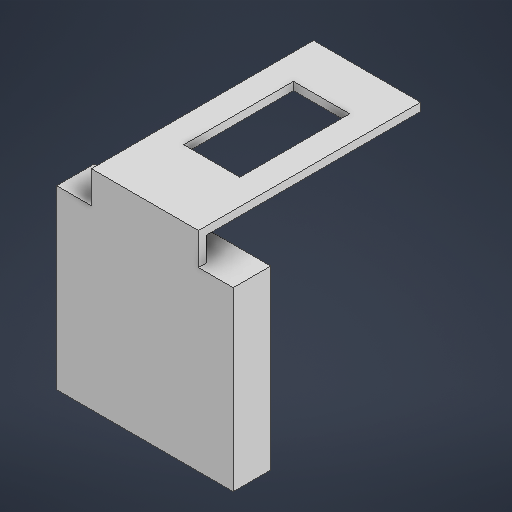
# Autodesk Inventor part: pan_base_holder
Saved by Autodesk Inventor 2026 (Build 300175000, 175)
## iProperties
Created: 2025-06-27
Part Number: pan_base_holder
Material: Generic
Document SubType Name: Modeling
Designer: user
Density: 1 g/cm^3
Appearance: Default
Author: user
Autodesk Inventor part; units mm, degrees
ref_plane "YZ Plane" through (0, 0, 0) normal (1, 0, 0) x (0, 1, 0)
ref_plane "XZ Plane" through (0, 0, 0) normal (0, 1, 0) x (-1, 0, 0)
ref_plane "XY Plane" through (0, 0, 0) normal (0, 0, 1) x (1, 0, 0)
sketch "Sketch1" plane through (0, 0, 0) normal (0, 0, 1) x (1, 0, 0)
  line L0 (-31, -31) -> (31, -31)
  line L1 (31, -31) -> (31, 31)
  line L2 (31, 31) -> (-31, 31)
  line L3 (-31, 31) -> (-31, -31)
  line L4 (-31, -31) -> (31, 31) construction
  line L5 (31, -31) -> (-31, 31) construction
  line L6 (-33, 33) -> (33, 33)
  line L7 (33, 33) -> (33, -33)
  line L8 (33, -33) -> (-33, -33)
  line L9 (-33, -33) -> (-33, 33)
  point P0 (0, 0)
  dimension "d0" = 62
  dimension "d1" = 62
  dimension "d2" = 2
  constraints: 20 end point, 4 parallel, 2 midpoint, 2 perpendicular, 1 horizontal, 3 other
  measures "d0" distance of L1.end L2.end
  measures "d1" distance of L0.end L1.end
  measures "d2" distance between parallel lines of L2 L6
extrude "Extrusion1" add sketch "Sketch1" along normal blind 2 contours L3 L2 L1 L0 | L6 L7 L8 L9
extrude "Extrusion2" add sketch "Sketch1" against normal blind 12
sketch "Sketch2" plane through (-33, 33, 2) normal (0, 1, 0) x (1, 0, 0)
  line L0 (13, 3) -> (53, 3)
  line L1 (53, 3) -> (53, 0)
  line L2 (53, 0) -> (13, 0)
  line L3 (13, 0) -> (13, 3)
  line L4 (0, 14) -> (0, 0) projected
  line L5 (0, 14) -> (66, 14) projected
  point P0 (33, 2)
  dimension "d7" = 40
  dimension "d8" = 3
  dimension "d9" = 13
  dimension "d10" = 11
  constraints: 8 end point, 2 parallel, 1 horizontal, 1 perpendicular
  measures "d7" distance of L1.end L2.end
  measures "d8" distance of L0.end L1.end
  measures "d9" distance between parallel lines of L4 L3
  measures "d10" distance between parallel lines of L5 L0
extrude "Extrusion3" add sketch "Sketch2" along normal blind 12
sketch "Sketch3" plane through (20, 33, -1) normal (0, 0, -1) x (-1, 0, 0)
  line L0 (40, 12) -> (0, 12) projected
  line L1 (40, 0) -> (40, 12) projected
  line L2 (0, 12) -> (40, 12)
  line L3 (40, 12) -> (40, 9)
  line L4 (40, 9) -> (0, 9)
  line L5 (0, 9) -> (0, 12)
  point P0 (20, -33)
  dimension "d13" = 3
  constraints: 8 end point, 2 parallel, 1 horizontal, 1 perpendicular, 1 point on line
  measures "d13" distance of L2.end L3.end
extrude "Extrusion4" add sketch "Sketch3" along normal blind 80
sketch "Sketch4" plane through (-20, 42, -1) normal (0, -1, 0) x (1, 0, 0)
  line L0 (30.5, -63) -> (9.5, -63)
  line L1 (9.5, -63) -> (9.5, -22)
  line L2 (9.5, -22) -> (30.5, -22)
  line L3 (30.5, -22) -> (30.5, -63)
  line L4 (40, 3) -> (40, -80) projected
  line L5 (0, 3) -> (40, 3) projected
  point P0 (20, 1)
  dimension "d16" = 21
  dimension "d17" = 41
  dimension "d18" = 9.5
  dimension "d19" = 25
  constraints: 8 end point, 2 parallel, 1 horizontal, 1 perpendicular
  measures "d16" distance of L0.start L0.end
  measures "d17" distance of L0.end L1.end
  measures "d18" distance between parallel lines of L4 L3
  measures "d19" distance between parallel lines of L2 L5
extrude "Extrusion5" cut sketch "Sketch4" against normal blind 80
body "Solid1"
